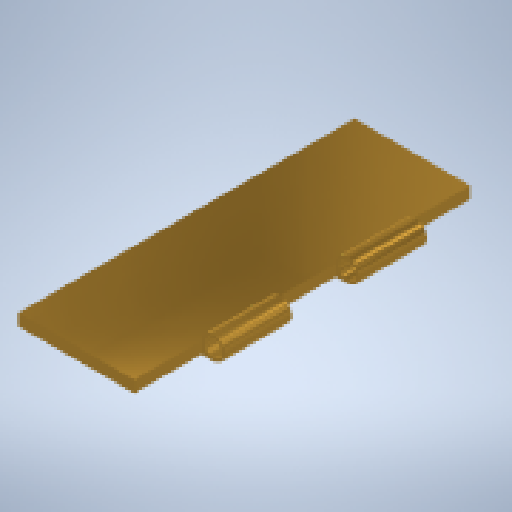
# Autodesk Inventor part: SchanierTeilB
Saved by Autodesk Inventor 2024 (Build 280153000, 153)
## iProperties
Created: 2023-11-30
Part Number: SchanierTeilB
Material: Generic
Document SubType Name: Modeling
Designer: Daniel Nussbaum
Density: 1 g/cm^3
Appearance: Default
Author: Daniel Nussbaum
Autodesk Inventor part; units mm, degrees
ref_plane "YZ Plane" through (0, 0, 0) normal (1, 0, 0) x (0, 1, 0)
ref_plane "XZ Plane" through (0, 0, 0) normal (0, 1, 0) x (-1, 0, 0)
ref_plane "XY Plane" through (0, 0, 0) normal (0, 0, 1) x (1, 0, 0)
sketch "Sketch1" plane through (0, 0, 0) normal (0, 0, 1) x (1, 0, 0)
  line L0 (0, 0) -> (-20, 0)
  line L1 (-20, 0) -> (-20, 2)
  line L2 (-20, 2) -> (0, 2)
  line L3 (0, 2) -> (0, 0)
  line L4 (0, 2) -> (2, 2)
  circle A0 centre (2, 2) radius 2
  line L5 (2, 0) -> (0, 0)
  dimension "d0" = 20
  dimension "d1" = 2
  dimension "d2" = 2
  constraints: 12 end point, 2 horizontal, 2 parallel, 2 point on circle, 1 centre point, 1 coincident, 1 collinear, 1 perpendicular
  measures "d0" distance of L1.end L2.end
  measures "d1" distance of L0.end L1.end
  measures "d2" distance of L2.end L4.end
extrude "Extrusion1" add sketch "Sketch1" along normal blind 58
sketch "Sketch2" plane through (-20, 2, 0) normal (0, 1, 0) x (1, 0, 0)
  line L0 (22, 0) -> (20, 0) projected
  line L1 (20, 0) -> (20, -58) projected
  line L2 (22, -58) -> (20, -58) projected
  line L3 (22, 0) -> (22, -58) projected
  line L4 (20, 0) -> (0, 0) projected
  line L5 (0, 0) -> (0, -58) projected
  line L6 (20, -58) -> (0, -58) projected
  line L7 (20, 0) -> (20, -58) projected
  line L8 (20, 0) -> (24, 0) projected
  line L9 (24, 0) -> (20, 0)
  line L10 (20, 0) -> (20, -11.6)
  line L11 (20, -11.6) -> (24, -11.6)
  line L12 (24, -11.6) -> (24, 0)
  line L13 (20, -11.6) -> (24, -11.6)
  line L14 (24, -11.6) -> (24, -23.2)
  line L15 (24, -23.2) -> (20, -23.2)
  line L16 (20, -23.2) -> (20, -11.6)
  line L17 (24, -23.2) -> (20, -23.2)
  line L18 (20, -23.2) -> (20, -34.8)
  line L19 (20, -34.8) -> (24, -34.8)
  line L20 (24, -34.8) -> (24, -23.2)
  line L21 (24, 0) -> (24, -58) projected
  line L22 (20, -34.8) -> (24, -34.8)
  line L23 (24, -34.8) -> (24, -46.4)
  line L24 (24, -46.4) -> (20, -46.4)
  line L25 (20, -46.4) -> (20, -34.8)
  line L26 (24, -46.4) -> (20, -46.4)
  line L27 (20, -46.4) -> (20, -58)
  line L28 (20, -58) -> (24, -58)
  line L29 (24, -58) -> (24, -46.4)
  dimension "d5" = 11.6
  dimension "d6" = 11.6
  dimension "d7" = 11.6
  dimension "d8" = 11.6
  constraints: 40 end point, 10 parallel, 5 horizontal, 5 perpendicular, 4 point on line
  measures "d5" distance of L10.end L9.end
  measures "d6" distance of L13.end L14.end
  measures "d7" distance of L18.end L17.end
  measures "d8" distance of L22.end L23.end
extrude "Extrusion2" cut sketch "Sketch2" along normal mid plane 4 contours L3 L11 L1 L0 | L8 L12 L11 L3 | L15 L20 L19 L3 | L3 L19 L1 L15 | L1 L24 L3 L2 | L24 L21 L28 L3
sketch "Sketch3" plane through (0, 0, 58) normal (0, 0, 1) x (1, 0, 0)
  arc A0 (2, 0) -> (0, 2) centre (2, 2) ccw projected
  line L0 (0, 2) -> (0, 0) projected
  line L1 (2, 0) -> (0, 0) projected
hole "Hole1" at (2, 2, 58) direction (0, 0, -1) diameter 3 end through all
body "Solid1"
